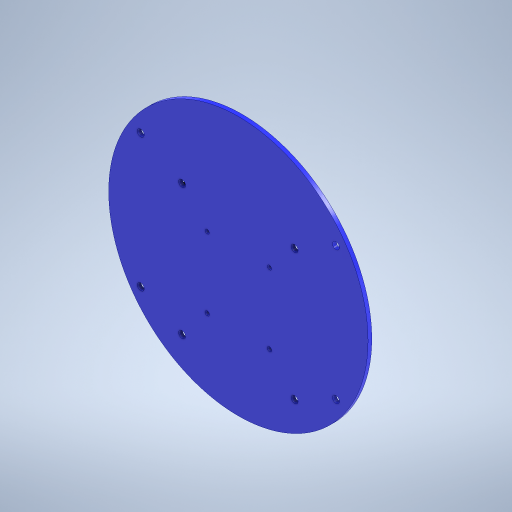
# Autodesk Inventor part: Alphabot_SUP
Saved by Autodesk Inventor 2023 (Build 270158030, 158C)
## iProperties
Created: 2022-07-21
Part Number: Alphabot_SUP
Material: Genérico
Document SubType Name: Modeling
Designer: luisn
Density: 1 g/cm^3
Appearance: Valor por defecto
Author: luisn
Autodesk Inventor part; units mm, degrees
ref_plane "YZ Plane" through (0, 0, 0) normal (1, 0, 0) x (0, 1, 0)
ref_plane "XZ Plane" through (0, 0, 0) normal (0, 1, 0) x (-1, 0, 0)
ref_plane "XY Plane" through (0, 0, 0) normal (0, 0, 1) x (1, 0, 0)
sketch "Boceto1" plane through (0, 0, 0) normal (0, 0, 1) x (1, 0, 0)
  circle A0 centre (0, 0) radius 55
  dimension "d0" = 110
  constraints: 1 centre point, 1 coincident
  measures "d0" diameter of A0
extrude "Extrusión1" add sketch "Boceto1" along normal blind 1.6
sketch "Boceto2" plane through (0, 0, 0) normal (0, 0, -1) x (-1, 0, 0)
  circle A0 centre (41.4, -28.25) radius 1.45
  line L0 (41.4, -28.25) -> (41.4, 0) construction
  line L1 (41.4, -28.25) -> (0, -28.25) construction
  line L2 (0, 0) -> (41.4, 0) construction
  circle A1 centre (0, 0) radius 55 construction
  line L3 (0, -28.25) -> (0, 0) construction
  line L4 (23.875, 0) -> (23.875, -37.0478) construction
  line L5 (23.875, -37.0478) -> (0, -37.0478) construction
  circle A2 centre (23.875, -37.0478) radius 1.45
  line L6 (23.875, -37.0478) -> (23.875, -49.5478) construction
  line L7 (23.875, 0) -> (23.875, 18.4522) construction
  circle A3 centre (23.875, 18.4522) radius 1.45
  line L8 (13.21, -23.89) -> (13.21, 6.11) construction
  circle A4 centre (13.21, -23.89) radius 0.925
  circle A5 centre (13.21, 6.11) radius 0.85
  line L9 (13.21, -23.89) -> (13.21, -53.39) construction
  dimension "d3" = 2.9
  dimension "d4" = 28.25
  dimension "d5" = 41.4
  dimension "d6" = 23.875
  dimension "d8" = 12.5
  dimension "d13" = 55.5
  dimension "d14" = 1.85
  dimension "d15" = 30
  dimension "d16" = 1.7
  dimension "d17" = 13.21
  dimension "d18" = 29.5
  constraints: 20 end point, 6 vertical, 5 centre point, 4 coincident, 3 point on line, 2 equal radius, 2 horizontal, 2 point on circle, 1 perpendicular
  measures "d3" diameter of A0
  measures "d4" distance of L0.start L0.end
  measures "d5" distance of L0.start L1.end
  measures "d6" distance of L4.end L5.end
  measures "d8" distance of L6.start L6.end
  measures "d13" distance of L4.end L7.end
  measures "d14" diameter of A4
  measures "d15" distance of L8.start L8.end
  measures "d16" diameter of A5
  measures "d17" distance between parallel lines of L3 L8
  measures "d18" distance of L9.start L9.end
extrude "Extrusión2" cut sketch "Boceto2" against normal blind 1.6 contours A0
mirror "Simetría1" about plane through (0, 0, 0) normal (0, 1, 0) of "Extrusión2"
mirror "Simetría2" about plane through (0, 0, 0) normal (1, 0, 0) of "Extrusión2", "Simetría1"
extrude "Extrusión3" cut sketch "Boceto2" against normal blind 1.6 contours A2 | A3 | A4 | A5
mirror "Simetría3" about plane through (0, 0, 0) normal (1, 0, 0) of "Extrusión3"
sketch "Boceto4" plane through (0, 0, 0) normal (0, 0, -1) x (-1, 0, 0)
  line L0 (21.375, -34.8978) -> (26.375, -34.8978)
  line L1 (26.375, -34.8978) -> (26.375, 16.2022)
  line L2 (26.375, 16.2022) -> (21.375, 16.2022)
  line L3 (21.375, 16.2022) -> (21.375, -34.8978)
  circle A0 centre (-23.875, 18.4522) radius 1.45 construction
  circle A1 centre (-13.21, -23.89) radius 0.925 construction
  circle A2 centre (-23.875, -37.0478) radius 1.45 construction
  circle A3 centre (-13.21, 6.11) radius 0.85 construction
  circle A4 centre (23.875, 18.4522) radius 1.45 construction
  circle A5 centre (13.21, -23.89) radius 0.925 construction
  circle A6 centre (23.875, -37.0478) radius 1.45 construction
  circle A7 centre (13.21, 6.11) radius 0.85 construction
  circle A8 centre (-41.4, 28.25) radius 1.45 construction
  circle A9 centre (-41.4, -28.25) radius 1.45 construction
  circle A10 centre (41.4, 28.25) radius 1.45 construction
  circle A11 centre (41.4, -28.25) radius 1.45 construction
  circle A12 centre (0, 0) radius 55 construction
  circle A13 centre (23.875, -37.0478) radius 1.45 construction
  circle A14 centre (23.875, 18.4522) radius 1.45 construction
  line L4 (23.875, -37.0478) -> (23.875, 18.4522) construction
  line L5 (-12.6, -49.14) -> (12.6, -49.14)
  line L6 (12.6, -49.14) -> (12.6, -44.03)
  line L7 (12.6, -44.03) -> (-12.6, -44.03)
  line L8 (-12.6, -44.03) -> (-12.6, -49.14)
  line L9 (0, 0) -> (0, -44.03) construction
  line L10 (0, -49.14) -> (0, -55) construction
  line L11 (-7.5, 19) -> (7.5, 19)
  line L12 (7.5, 19) -> (7.5, 21.5)
  line L13 (7.5, 21.5) -> (-7.5, 21.5)
  line L14 (-7.5, 21.5) -> (-7.5, 19)
  line L15 (0, 0) -> (0, 19) construction
  line L16 (0, 21.5) -> (0, 55) construction
  line L17 (-30.4995, -4.8454) -> (-22.0995, -4.8454)
  line L18 (-22.0995, -4.8454) -> (-22.0995, 5.3046)
  line L19 (-22.0995, 5.3046) -> (-30.4995, 5.3046)
  line L20 (-30.4995, 5.3046) -> (-30.4995, -4.8454)
  line L21 (-26.2995, 5.3046) -> (-26.2995, 48.3046) construction
  circle A15 centre (0, 0) radius 55 construction
  line L22 (-30.4995, 0.2296) -> (-54.9995, 0.2296) construction
  line L23 (-14.5995, -17.78) -> (-10.2495, -17.78)
  line L24 (-10.2495, -17.78) -> (-10.2495, -7.98)
  line L25 (-10.2495, -7.98) -> (-14.5995, -7.98)
  line L26 (-14.5995, -7.98) -> (-14.5995, -17.78)
  line L27 (2.125, -20.3978) -> (14.875, -20.3978)
  line L28 (14.875, -20.3978) -> (14.875, -12.6478)
  line L29 (14.875, -12.6478) -> (2.125, -12.6478)
  line L30 (2.125, -12.6478) -> (2.125, -20.3978)
  circle A16 centre (-31.2995, -24.8454) radius 3.125
  circle A17 centre (-21.2995, -24.8454) radius 3.125
  line L31 (-21.2995, -24.8454) -> (-31.2995, -24.8454) construction
  line L32 (-26.2995, -4.8454) -> (-26.2995, -24.8454) construction
  point P0 (23.875, -34.8978)
  dimension "d19" = 51.1
  dimension "d20" = 5
  dimension "d21" = 2.15
  dimension "d24" = 25.2
  dimension "d25" = 5.11
  dimension "d26" = 5.86
  dimension "d27" = 15
  dimension "d28" = 2.5
  dimension "d29" = 33.5
  dimension "d30" = 10.15
  dimension "d31" = 8.4
  dimension "d32" = 43
  dimension "d33" = 24.5
  dimension "d34" = 9.8
  dimension "d35" = 4.35
  dimension "d36" = 26.25
  dimension "d37" = 7.5
  dimension "d38" = 12.75
  dimension "d39" = 7.75
  dimension "d40" = 14.5
  dimension "d41" = 6.5
  dimension "d50" = 6.25
  dimension "d51" = 10
  dimension "d52" = 20
  constraints: 66 end point, 12 parallel, 9 midpoint, 8 horizontal, 7 vertical, 6 perpendicular, 4 point on circle, 2 centre point, 1 equal radius, 1 point on line
  measures "d19" distance of L2.end L0.start
  measures "d20" distance of L1.end L2.end
  measures "d21" distance from line of A6.centre L0
  measures "d24" distance of L6.end L7.end
  measures "d25" distance of L7.end L5.start
  measures "d26" distance of L10.start L10.end
  measures "d27" distance of L11.start L11.end
  measures "d28" distance of L11.end L12.end
  measures "d29" distance of L16.start L16.end
  measures "d30" distance of L19.end L17.start
  measures "d31" distance of L18.end L19.end
  measures "d32" distance of L21.start L21.end
  measures "d33" distance of L22.start L22.end
  measures "d34" distance of L25.end L23.start
  measures "d35" distance between parallel lines of L26 L24
  measures "d36" distance between parallel lines of L23 L7
  measures "d37" distance between parallel lines of L18 L26
  measures "d38" distance of L28.end L29.end
  measures "d39" distance of L29.end L27.start
  measures "d40" distance between parallel lines of L0 L27
  measures "d41" distance between parallel lines of L3 L28
  measures "d50" diameter of A16
  measures "d51" distance of L31.start L31.end
  measures "d52" distance between parallel lines of L31 L17
extrude "Extrusión4" add sketch "Boceto4" along normal blind 13.35 separate body contours L3 L2 L1 L0
extrude "Extrusión5" add sketch "Boceto4" along normal blind 4.3 separate body contours L8 L7 L6 L5
extrude "Extrusión6" add sketch "Boceto4" along normal blind 4.5 separate body contours L20 L19 L18 L17
extrude "Extrusión7" add sketch "Boceto4" along normal blind 0.85 separate body contours L26 L25 L24 L23
extrude "Extrusión8" add sketch "Boceto4" along normal blind 2.45 separate body contours L30 L29 L28 L27
extrude "Extrusión9" add sketch "Boceto4" along normal blind 5.75 separate body contours A16 | A17
